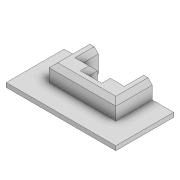
# Autodesk Inventor part: millmax_solder_rig
Saved by Autodesk Inventor 2021 (Build 250183000, 183)
## iProperties
Created: 2021-05-18
Part Number: millmax_solder_rig
Material: Generic
Document SubType Name: Modeling
Designer: Daniel
Density: 1 g/cm^3
Appearance: Default
Author: Daniel
Autodesk Inventor part; units mm, degrees
ref_plane "YZ Plane" through (0, 0, 0) normal (1, 0, 0) x (0, 1, 0)
ref_plane "XZ Plane" through (0, 0, 0) normal (0, 1, 0) x (-1, 0, 0)
ref_plane "XY Plane" through (0, 0, 0) normal (0, 0, 1) x (1, 0, 0)
sketch "Sketch1" plane through (0, 0, 0) normal (0, 1, 0) x (-1, 0, 0)
  line L0 (0, 0) -> (19.1, 0)
  line L1 (19.1, 0) -> (19.1, -10)
  line L2 (19.1, -10) -> (0, -10)
  line L3 (0, -10) -> (0, 0)
  line L4 (12.55, -10) -> (6.55, -10)
  line L5 (6.55, -10) -> (6.55, -6)
  line L6 (6.55, -6) -> (12.55, -6)
  line L7 (12.55, -6) -> (12.55, -10)
  line L8 (0, 0) -> (-6, 0)
  line L9 (-6, 0) -> (-6, -17)
  line L10 (-6, -17) -> (0, -17)
  line L11 (0, -17) -> (0, 0)
  line L12 (19.1, 0) -> (25.1, 0)
  line L13 (25.1, 0) -> (25.1, -17)
  line L14 (25.1, -17) -> (19.1, -17)
  line L15 (19.1, -17) -> (19.1, 0)
  point P0 (9.55, -6)
  point P1 (9.55, 0)
  point P2 (6.55, -10)
  point P3 (0, -10)
  dimension "d0" = 6
  dimension "d1" = 19.1
  dimension "d2" = 4
  dimension "d3" = 10
  dimension "d6" = 6
  dimension "d7" = 6
  dimension "d8" = 17
  dimension "d20" = 7
  constraints: 32 end point, 8 parallel, 4 horizontal, 4 perpendicular, 2 midpoint, 1 collinear, 1 point on line, 1 vertical alignment
  measures "d0" distance between parallel lines of L5 L7
  measures "d1" distance between parallel lines of L3 L1
  measures "d2" distance of L6.end L4.start
  measures "d3" distance of L0.end L1.end
  measures "d6" distance of L13.end L14.end
  measures "d7" distance of L9.end L10.end
  measures "d8" distance of L12.end L13.end
  measures "d20" distance between parallel lines of L14 L2
extrude "Extrusion1" add sketch "Sketch1" along normal blind 10 contours L0 L1 L2 L7 L6 L5 L3 | L3 L11 L10 L9 L8 | L12 L13 L14 L15 L1
sketch "Sketch2" plane through (0, 0, 0) normal (0, -1, 0) x (1, 0, 0)
  line L0 (-25.1, 0) -> (6, 0) projected
  line L1 (-25.1, -17) -> (-25.1, 0) projected
  line L2 (-19.1, -17) -> (-25.1, -17) projected
  line L3 (-19.1, -10) -> (-19.1, -17) projected
  line L4 (-12.55, -10) -> (-19.1, -10) projected
  line L5 (-12.55, -6) -> (-12.55, -10) projected
  line L6 (-6.55, -6) -> (-12.55, -6) projected
  line L7 (-6.55, -10) -> (-6.55, -6) projected
  line L8 (0, -10) -> (-6.55, -10) projected
  line L9 (0, -17) -> (0, -10) projected
  line L10 (6, -17) -> (0, -17) projected
  line L11 (6, 0) -> (6, -17) projected
  line L12 (6, -17) -> (16, -17)
  line L13 (16, -17) -> (16, 10)
  line L14 (16, 10) -> (-35.1, 10)
  line L15 (-35.1, 10) -> (-35.1, -17)
  line L16 (-35.1, -17) -> (-25.1, -17)
  point P0 (0, 0)
  dimension "d9" = 10
  dimension "d10" = 10
  dimension "d11" = 10
  constraints: 10 end point, 4 perpendicular, 1 horizontal, 1 point on line
  measures "d9" distance between parallel lines of L1 L15
  measures "d10" distance between parallel lines of L14 L0
  measures "d11" distance between parallel lines of L11 L13
extrude "Extrusion2" add sketch "Sketch2" against normal blind 2 contours L1 L16 L15 L14 L13 L12 L11 L0
chamfer "Chamfer1" distance 2 angle 45 7 edges at (-19.1, 10, -13.5) (-15.825, 10, -10) (-9.55, 10, -6) (-6.55, 10, -8) (0, 10, -13.5) (-3.275, 10, -10) (-12.55, 10, -8)
chamfer "Chamfer2" distance 2 angle 45 3 edges at (6, 10, -8.5) (-9.55, 10, 0) (-25.1, 10, -8.5)
body "Solid1"
